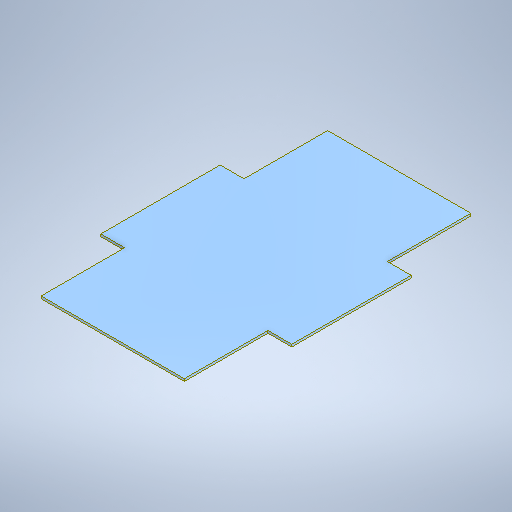
# Autodesk Inventor part: нижняя плита
Saved by Autodesk Inventor 2025 (Build 290162000, 162)
## iProperties
Created: 2025-01-21
Part Number: нижняя плита
Material: Типовые
Document SubType Name: Modeling
Designer: volko
Density: 1 g/cm^3
Appearance: По умолчанию
Author: volko
Autodesk Inventor part; units mm, degrees
ref_plane "YZ Plane" through (0, 0, 0) normal (1, 0, 0) x (0, 1, 0)
ref_plane "XZ Plane" through (0, 0, 0) normal (0, 1, 0) x (-1, 0, 0)
ref_plane "XY Plane" through (0, 0, 0) normal (0, 0, 1) x (1, 0, 0)
sketch "Эскиз1" plane through (0, 0, 0) normal (0, 1, 0) x (-1, 0, 0)
  line L0 (0, 300) -> (150, 300)
  line L1 (150, 300) -> (150, 125)
  line L2 (150, 125) -> (200, 125)
  line L3 (200, 125) -> (200, 0)
  line L4 (0, 300) -> (0, 0)
  line L5 (0, 0) -> (200, 0)
  line L6 (0, 300) -> (-150, 300)
  line L7 (-150, 300) -> (-150, 125)
  line L8 (-150, 125) -> (-200, 125)
  line L9 (-200, 125) -> (-200, 0)
  line L10 (0, -300) -> (150, -300)
  line L11 (150, -300) -> (150, -125)
  line L12 (150, -125) -> (200, -125)
  line L13 (200, -125) -> (200, 0)
  line L14 (-200, -125) -> (-200, 0)
  line L15 (-150, -125) -> (-200, -125)
  line L16 (-150, -300) -> (-150, -125)
  line L17 (0, -300) -> (-150, -300)
  point P0 (175, -125)
  point P1 (175, 125)
  dimension "d1" = 400
  dimension "d3" = 300
  dimension "d6" = 600
  dimension "d7" = 250
  constraints: 36 end point, 11 symmetric about line, 3 perpendicular, 2 midpoint, 2 point on line, 1 vertical
  measures "d1" distance between parallel lines of L9 L3
  measures "d3" distance between parallel lines of L7 L1
  measures "d6" distance between parallel lines of L6 L17
  measures "d7" distance of point (175, -125) point (175, 125)
extrude "Выдавливание1" add sketch "Эскиз1" along normal blind 5
